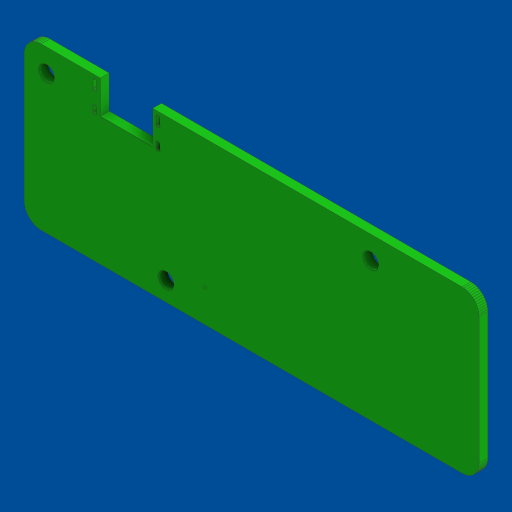
# Autodesk Inventor part: PCB
Saved by Autodesk Inventor 2023.2 (Build 272271000, 271)
## iProperties
Created: 2023-06-14
Part Number: PCB
Material: Generic
Document SubType Name: Modeling
Designer: samdi
Density: 1 g/cm^3
Appearance: Default
Author: samdi
Autodesk Inventor part; units mm, degrees
ref_plane "YZ Plane" through (0, 0, 0) normal (1, 0, 0) x (0, 1, 0)
ref_plane "XZ Plane" through (0, 0, 0) normal (0, 1, 0) x (-1, 0, 0)
ref_plane "XY Plane" through (0, 0, 0) normal (0, 0, 1) x (1, 0, 0)
sketch "Sketch1" plane through (0, 0, 0) normal (0, 0, 1) x (1, 0, 0)
  line L0 (-1.2818, 20.3685) -> (-1.1938, 20.3021)
  line L1 (-1.3879, 20.3987) -> (-1.2818, 20.3685)
  line L2 (-1.4976, 20.3885) -> (-1.3879, 20.3987)
  line L3 (-1.5963, 20.3394) -> (-1.4976, 20.3885)
  line L4 (-1.6706, 20.2579) -> (-1.5963, 20.3394)
  line L5 (-1.1938, 20.3021) -> (-1.1358, 20.2084)
  line L6 (-1.1605, 19.1421) -> (-1.2348, 19.0606)
  line L7 (-1.2348, 19.0606) -> (-1.3335, 19.0115)
  circle A0 centre (6.8571, 2.31) radius 0.15
  circle A1 centre (0, 0) radius 1.35
  line L8 (-1.1156, 19.3) -> (-1.1207, 19.2449)
  line L9 (-1.1156, 20.1) -> (-1.1156, 19.3)
  line L10 (-1.1358, 20.2084) -> (-1.1156, 20.1)
  line L11 (-1.1938, 20.3021) -> (-1.1358, 20.2084)
  line L12 (-1.2818, 20.3685) -> (-1.1938, 20.3021)
  line L13 (-1.3879, 20.3987) -> (-1.2818, 20.3685)
  line L14 (-1.1207, 19.2449) -> (-1.1605, 19.1421)
  circle A2 centre (6.8571, 2.31) radius 0.15
  circle A3 centre (-21, 21) radius 1.35
  line L15 (-22.6676, 24.9248) -> (-22.3359, 24.9811)
  line L16 (-1.1361, 24.2084) -> (-1.1159, 24.1)
  line L17 (-1.7159, 24.1) -> (-1.7107, 24.1551)
  line L18 (-1.7159, 22.9) -> (-1.7159, 24.1)
  line L19 (-1.6956, 22.7916) -> (-1.7159, 22.9)
  line L20 (-1.6376, 22.6979) -> (-1.6956, 22.7916)
  line L21 (-1.1159, 24.1) -> (-1.1159, 22.9)
  line L22 (-1.1159, 22.9) -> (-1.121, 22.8449)
  line L23 (-1.121, 22.8449) -> (-1.1608, 22.7421)
  line L24 (-1.7107, 24.1551) -> (-1.6709, 24.2579)
  line L25 (-1.1941, 24.3021) -> (-1.1361, 24.2084)
  line L26 (-1.2821, 24.3685) -> (-1.1941, 24.3021)
  line L27 (-1.3882, 24.3987) -> (-1.2821, 24.3685)
  line L28 (-1.4979, 24.3885) -> (-1.3882, 24.3987)
  line L29 (-1.5966, 24.3394) -> (-1.4979, 24.3885)
  line L30 (-24.7029, -1.6803) -> (-24.8316, -1.3695)
  line L31 (-24.8316, -1.3695) -> (-24.9248, -1.0462)
  line L32 (-24.9248, -1.0462) -> (-24.9811, -0.7146)
  line L33 (-24.9811, -0.7146) -> (-25, -0.3787)
  line L34 (-25, -0.3787) -> (-25, 22)
  line L35 (-25, 22) -> (-24.9811, 22.3359)
  line L36 (-24.9811, 22.3359) -> (-24.9248, 22.6676)
  line L37 (-24.5402, -1.9748) -> (-24.7029, -1.6803)
  line L38 (-22.9908, 24.8316) -> (-22.6676, 24.9248)
  line L39 (-23.3017, 24.7029) -> (-22.9908, 24.8316)
  line L40 (-23.5961, 24.5402) -> (-23.3017, 24.7029)
  line L41 (-23.8705, 24.3455) -> (-23.5961, 24.5402)
  line L42 (-24.1213, 24.1213) -> (-23.8705, 24.3455)
  line L43 (-24.3455, 23.8705) -> (-24.1213, 24.1213)
  line L44 (-24.5402, 23.5961) -> (-24.3455, 23.8705)
  line L45 (-24.7029, 23.3017) -> (-24.5402, 23.5961)
  line L46 (-24.8316, 22.9908) -> (-24.7029, 23.3017)
  line L47 (-24.9248, 22.6676) -> (-24.8316, 22.9908)
  line L48 (-12.8462, 22.7916) -> (-12.8665, 22.9)
  line L49 (-12.2665, 22.9) -> (-12.2716, 22.8449)
  line L50 (-12.8665, 22.9) -> (-12.8665, 24.1)
  line L51 (-12.2665, 24.1) -> (-12.2665, 22.9)
  line L52 (-12.8665, 24.1) -> (-12.8613, 24.1551)
  line L53 (-12.2867, 24.2084) -> (-12.2665, 24.1)
  line L54 (-12.8613, 24.1551) -> (-12.8215, 24.2579)
  line L55 (-12.3447, 24.3021) -> (-12.2867, 24.2084)
  line L56 (-12.8215, 24.2579) -> (-12.7472, 24.3394)
  line L57 (-12.4327, 24.3685) -> (-12.3447, 24.3021)
  line L58 (-12.5388, 24.3987) -> (-12.4327, 24.3685)
  line L59 (-12.6485, 24.3885) -> (-12.5388, 24.3987)
  line L60 (-12.7472, 24.3394) -> (-12.6485, 24.3885)
  line L61 (-12.2716, 22.8449) -> (-12.3114, 22.7421)
  line L62 (-12.7882, 22.6979) -> (-12.8462, 22.7916)
  line L63 (-12.3114, 22.7421) -> (-12.3857, 22.6606)
  line L64 (-12.7002, 22.6315) -> (-12.7882, 22.6979)
  line L65 (-12.3857, 22.6606) -> (-12.4844, 22.6115)
  line L66 (-12.5941, 22.6013) -> (-12.7002, 22.6315)
  line L67 (-12.4844, 22.6115) -> (-12.5941, 22.6013)
  line L68 (-1.7104, 20.1551) -> (-1.6706, 20.2579)
  line L69 (-1.7156, 20.1) -> (-1.7104, 20.1551)
  line L70 (-1.5493, 19.0315) -> (-1.6373, 19.0979)
  line L71 (-1.7156, 19.3) -> (-1.7156, 20.1)
  line L72 (-1.6953, 19.1916) -> (-1.7156, 19.3)
  line L73 (-1.6373, 19.0979) -> (-1.6953, 19.1916)
  line L74 (-1.1605, 19.1421) -> (-1.2348, 19.0606)
  line L75 (-1.2348, 19.0606) -> (-1.3335, 19.0115)
  line L76 (-1.3335, 19.0115) -> (-1.4432, 19.0013)
  line L77 (-1.4432, 19.0013) -> (-1.5493, 19.0315)
  line L78 (-1.1207, 19.2449) -> (-1.1605, 19.1421)
  line L79 (-1.1608, 22.7421) -> (-1.2351, 22.6606)
  line L80 (-1.2351, 22.6606) -> (-1.3338, 22.6115)
  line L81 (-1.3338, 22.6115) -> (-1.4435, 22.6013)
  line L82 (-1.4435, 22.6013) -> (-1.5496, 22.6315)
  line L83 (-1.5496, 22.6315) -> (-1.6376, 22.6979)
  line L84 (-1.1159, 24.1) -> (-1.1159, 22.9)
  line L85 (-1.1159, 22.9) -> (-1.121, 22.8449)
  line L86 (-1.1361, 24.2084) -> (-1.1159, 24.1)
  line L87 (-1.121, 22.8449) -> (-1.1608, 22.7421)
  line L88 (-1.1941, 24.3021) -> (-1.1361, 24.2084)
  line L89 (-1.2821, 24.3685) -> (-1.1941, 24.3021)
  line L90 (-1.3335, 19.0115) -> (-1.4432, 19.0013)
  line L91 (-1.4979, 24.3885) -> (-1.3882, 24.3987)
  line L92 (-1.5966, 24.3394) -> (-1.4979, 24.3885)
  line L93 (-1.6709, 24.2579) -> (-1.5966, 24.3394)
  line L94 (-1.3882, 24.3987) -> (-1.2821, 24.3685)
  line L95 (-1.4976, 20.3885) -> (-1.3879, 20.3987)
  line L96 (-1.5963, 20.3394) -> (-1.4976, 20.3885)
  line L97 (-1.4432, 19.0013) -> (-1.5493, 19.0315)
  line L98 (-1.6706, 20.2579) -> (-1.5963, 20.3394)
  line L99 (-1.7104, 20.1551) -> (-1.6706, 20.2579)
  line L100 (-1.5493, 19.0315) -> (-1.6373, 19.0979)
  line L101 (-1.6373, 19.0979) -> (-1.6953, 19.1916)
  line L102 (-1.7156, 19.3) -> (-1.7156, 20.1)
  line L103 (-1.6953, 19.1916) -> (-1.7156, 19.3)
  line L104 (-1.7156, 20.1) -> (-1.7104, 20.1551)
  line L105 (-1.6956, 22.7916) -> (-1.7159, 22.9)
  line L106 (-1.6709, 24.2579) -> (-1.5966, 24.3394)
  line L107 (-1.5496, 22.6315) -> (-1.6376, 22.6979)
  line L108 (-1.4435, 22.6013) -> (-1.5496, 22.6315)
  line L109 (-1.3338, 22.6115) -> (-1.4435, 22.6013)
  line L110 (-1.2351, 22.6606) -> (-1.3338, 22.6115)
  line L111 (-1.1608, 22.7421) -> (-1.2351, 22.6606)
  line L112 (-1.1156, 19.3) -> (-1.1207, 19.2449)
  line L113 (-1.1156, 20.1) -> (-1.1156, 19.3)
  line L114 (-1.1358, 20.2084) -> (-1.1156, 20.1)
  line L115 (-2.3912, 25) -> (1.7088, 25)
  circle A4 centre (0, 0) radius 1.35
  line L116 (-12.8215, 20.2579) -> (-12.7472, 20.3394)
  line L117 (-12.8613, 20.1551) -> (-12.8215, 20.2579)
  line L118 (-2.3912, 25) -> (1.7088, 25)
  line L119 (-2.3912, 19.2) -> (-2.3912, 25)
  line L120 (-2.3912, 19.2) -> (-2.3912, 25)
  line L121 (-11.5911, 19.2) -> (-2.3912, 19.2)
  line L122 (-11.5911, 19.2) -> (-2.3912, 19.2)
  line L123 (-11.5911, 25) -> (-11.5911, 19.2)
  line L124 (-11.5911, 25) -> (-11.5911, 19.2)
  line L125 (-12.7472, 24.3394) -> (-12.6485, 24.3885)
  line L126 (-12.3114, 22.7421) -> (-12.3857, 22.6606)
  line L127 (-12.3857, 22.6606) -> (-12.4844, 22.6115)
  line L128 (-12.4844, 22.6115) -> (-12.5941, 22.6013)
  line L129 (-12.5941, 22.6013) -> (-12.7002, 22.6315)
  line L130 (-12.7002, 22.6315) -> (-12.7882, 22.6979)
  line L131 (-12.7882, 22.6979) -> (-12.8462, 22.7916)
  line L132 (-12.8462, 22.7916) -> (-12.8665, 22.9)
  line L133 (-12.8665, 22.9) -> (-12.8665, 24.1)
  line L134 (-12.8665, 24.1) -> (-12.8613, 24.1551)
  line L135 (-12.8613, 24.1551) -> (-12.8215, 24.2579)
  line L136 (-12.2867, 24.2084) -> (-12.2665, 24.1)
  line L137 (-12.2665, 24.1) -> (-12.2665, 22.9)
  line L138 (-12.2665, 22.9) -> (-12.2716, 22.8449)
  line L139 (-12.2716, 22.8449) -> (-12.3114, 22.7421)
  line L140 (-12.8462, 19.1916) -> (-12.8665, 19.3)
  line L141 (-12.8665, 19.3) -> (-12.8665, 20.1)
  line L142 (-1.7107, 24.1551) -> (-1.6709, 24.2579)
  line L143 (-1.7159, 24.1) -> (-1.7107, 24.1551)
  line L144 (-1.7159, 22.9) -> (-1.7159, 24.1)
  line L145 (-1.6376, 22.6979) -> (-1.6956, 22.7916)
  line L146 (-12.2867, 20.2084) -> (-12.2665, 20.1)
  line L147 (-12.2665, 20.1) -> (-12.2665, 19.3)
  line L148 (-12.3447, 20.3021) -> (-12.2867, 20.2084)
  line L149 (-12.2665, 19.3) -> (-12.2716, 19.2449)
  line L150 (-12.2716, 19.2449) -> (-12.3114, 19.1421)
  line L151 (-12.4327, 20.3685) -> (-12.3447, 20.3021)
  line L152 (-12.5388, 20.3987) -> (-12.4327, 20.3685)
  line L153 (-12.6485, 20.3885) -> (-12.5388, 20.3987)
  line L154 (-12.8665, 20.1) -> (-12.8613, 20.1551)
  line L155 (-12.7472, 20.3394) -> (-12.6485, 20.3885)
  line L156 (-12.6485, 20.3885) -> (-12.5388, 20.3987)
  line L157 (-12.7472, 20.3394) -> (-12.6485, 20.3885)
  line L158 (-12.4327, 20.3685) -> (-12.3447, 20.3021)
  line L159 (-12.8215, 20.2579) -> (-12.7472, 20.3394)
  line L160 (-12.3447, 20.3021) -> (-12.2867, 20.2084)
  line L161 (-12.8613, 20.1551) -> (-12.8215, 20.2579)
  line L162 (-12.2867, 20.2084) -> (-12.2665, 20.1)
  line L163 (-12.8665, 20.1) -> (-12.8613, 20.1551)
  line L164 (-12.8665, 19.3) -> (-12.8665, 20.1)
  line L165 (-12.2665, 20.1) -> (-12.2665, 19.3)
  line L166 (-12.2665, 19.3) -> (-12.2716, 19.2449)
  line L167 (-12.5388, 20.3987) -> (-12.4327, 20.3685)
  line L168 (-12.8462, 19.1916) -> (-12.8665, 19.3)
  line L169 (-12.7882, 19.0979) -> (-12.8462, 19.1916)
  line L170 (-12.7002, 19.0315) -> (-12.7882, 19.0979)
  line L171 (-12.5941, 19.0013) -> (-12.7002, 19.0315)
  line L172 (-12.4844, 19.0115) -> (-12.5941, 19.0013)
  line L173 (-12.3857, 19.0606) -> (-12.4844, 19.0115)
  line L174 (-12.3114, 19.1421) -> (-12.3857, 19.0606)
  line L175 (-12.2716, 19.2449) -> (-12.3114, 19.1421)
  line L176 (-15.0912, 25) -> (-11.5911, 25)
  line L177 (-22, 25) -> (-15.0912, 25)
  line L178 (-22.3359, 24.9811) -> (-22, 25)
  line L179 (-12.3447, 24.3021) -> (-12.2867, 24.2084)
  line L180 (-12.3114, 19.1421) -> (-12.3857, 19.0606)
  line L181 (-12.4327, 24.3685) -> (-12.3447, 24.3021)
  line L182 (-12.3857, 19.0606) -> (-12.4844, 19.0115)
  line L183 (-12.4844, 19.0115) -> (-12.5941, 19.0013)
  line L184 (-12.6485, 24.3885) -> (-12.5388, 24.3987)
  line L185 (-12.5941, 19.0013) -> (-12.7002, 19.0315)
  line L186 (-12.7002, 19.0315) -> (-12.7882, 19.0979)
  line L187 (-12.7882, 19.0979) -> (-12.8462, 19.1916)
  line L188 (-12.8215, 24.2579) -> (-12.7472, 24.3394)
  line L189 (-15.0912, 25) -> (-11.5911, 25)
  line L190 (-22, 25) -> (-15.0912, 25)
  circle A5 centre (-21, 21) radius 1.35
  line L191 (-12.5388, 24.3987) -> (-12.4327, 24.3685)
  line L192 (-22.3359, 24.9811) -> (-22, 25)
  line L193 (-22.6676, 24.9248) -> (-22.3359, 24.9811)
  line L194 (-22.9908, 24.8316) -> (-22.6676, 24.9248)
  line L195 (-23.5961, 24.5402) -> (-23.3017, 24.7029)
  line L196 (-23.3017, 24.7029) -> (-22.9908, 24.8316)
  line L197 (-23.8705, 24.3455) -> (-23.5961, 24.5402)
  line L198 (-24.1213, 24.1213) -> (-23.8705, 24.3455)
  line L199 (-24.5402, 23.5961) -> (-24.3455, 23.8705)
  line L200 (-24.7029, 23.3017) -> (-24.5402, 23.5961)
  line L201 (-24.3455, 23.8705) -> (-24.1213, 24.1213)
  line L202 (-25, -0.3787) -> (-25, 22)
  line L203 (-25, 22) -> (-24.9811, 22.3359)
  line L204 (-24.9811, 22.3359) -> (-24.9248, 22.6676)
  line L205 (-24.8316, 22.9908) -> (-24.7029, 23.3017)
  line L206 (-24.9248, 22.6676) -> (-24.8316, 22.9908)
  line L207 (-23.3017, -3.0816) -> (-23.5961, -2.9189)
  line L208 (-23.5961, -2.9189) -> (-23.8705, -2.7242)
  line L209 (-23.8705, -2.7242) -> (-24.1213, -2.5)
  line L210 (-24.1213, -2.5) -> (-24.3455, -2.2491)
  line L211 (-24.3455, -2.2491) -> (-24.5402, -1.9748)
  line L212 (-24.3455, -2.2491) -> (-24.5402, -1.9748)
  line L213 (-24.1213, -2.5) -> (-24.3455, -2.2491)
  line L214 (-23.8705, -2.7242) -> (-24.1213, -2.5)
  line L215 (52, -3.3787) -> (-22, -3.3787)
  line L216 (52, -3.3787) -> (-22, -3.3787)
  line L217 (1.7088, 25) -> (52, 25)
  line L218 (1.7088, 25) -> (52, 25)
  circle A6 centre (36, 21) radius 1.35
  line L219 (52, 25) -> (52.3359, 24.9811)
  line L220 (52.6676, 24.9248) -> (52.9908, 24.8316)
  line L221 (52.9908, 24.8316) -> (53.3017, 24.7029)
  line L222 (53.8705, 24.3455) -> (54.1213, 24.1213)
  line L223 (54.3455, 23.8705) -> (54.5402, 23.5961)
  line L224 (54.8317, 22.9908) -> (54.9248, 22.6676)
  line L225 (54.8317, 22.9908) -> (54.9248, 22.6676)
  line L226 (52.3359, -3.3598) -> (52, -3.3787)
  line L227 (52, 25) -> (52.3359, 24.9811)
  line L228 (52.3359, 24.9811) -> (52.6676, 24.9248)
  line L229 (52.3359, 24.9811) -> (52.6676, 24.9248)
  line L230 (52.6676, 24.9248) -> (52.9908, 24.8316)
  line L231 (53.3017, 24.7029) -> (53.5961, 24.5402)
  line L232 (53.3017, 24.7029) -> (53.5961, 24.5402)
  line L233 (53.5961, 24.5402) -> (53.8705, 24.3455)
  line L234 (54.9811, 22.3359) -> (55, 22)
  line L235 (54.1213, 24.1213) -> (54.3455, 23.8705)
  line L236 (54.9248, 22.6676) -> (54.9811, 22.3359)
  line L237 (54.5402, 23.5961) -> (54.7029, 23.3017)
  line L238 (54.7029, 23.3017) -> (54.8317, 22.9908)
  line L239 (52.9908, 24.8316) -> (53.3017, 24.7029)
  line L240 (53.5961, 24.5402) -> (53.8705, 24.3455)
  line L241 (55, 22) -> (55, -0.3787)
  line L242 (53.5961, -2.9189) -> (53.3017, -3.0816)
  line L243 (53.5961, -2.9189) -> (53.3017, -3.0816)
  line L244 (54.3455, -2.2491) -> (54.1213, -2.5)
  line L245 (54.8317, -1.3695) -> (54.7029, -1.6803)
  line L246 (54.9811, -0.7146) -> (54.9248, -1.0462)
  line L247 (54.9248, -1.0462) -> (54.8317, -1.3695)
  line L248 (54.7029, -1.6803) -> (54.5402, -1.9748)
  line L249 (54.5402, -1.9748) -> (54.3455, -2.2491)
  line L250 (54.1213, -2.5) -> (53.8705, -2.7242)
  line L251 (53.3017, -3.0816) -> (52.9908, -3.2103)
  line L252 (52.9908, -3.2103) -> (52.6676, -3.3035)
  line L253 (52.3359, -3.3598) -> (52, -3.3787)
  line L254 (55, -0.3787) -> (54.9811, -0.7146)
  line L255 (-22, -3.3787) -> (-22.3359, -3.3598)
  line L256 (-22.6676, -3.3035) -> (-22.9908, -3.2103)
  line L257 (-22.9908, -3.2103) -> (-23.3017, -3.0816)
  line L258 (-22.3359, -3.3598) -> (-22.6676, -3.3035)
  line L259 (-22, -3.3787) -> (-22.3359, -3.3598)
  line L260 (-23.5961, -2.9189) -> (-23.8705, -2.7242)
  line L261 (-23.3017, -3.0816) -> (-23.5961, -2.9189)
  line L262 (-22.9908, -3.2103) -> (-23.3017, -3.0816)
  line L263 (-22.6676, -3.3035) -> (-22.9908, -3.2103)
  line L264 (-22.3359, -3.3598) -> (-22.6676, -3.3035)
  circle A7 centre (36, 21) radius 1.35
  line L265 (52.6676, -3.3035) -> (52.3359, -3.3598)
  line L266 (53.3017, -3.0816) -> (52.9908, -3.2103)
  line L267 (53.8705, -2.7242) -> (53.5961, -2.9189)
  line L268 (55, -0.3787) -> (54.9811, -0.7146)
  line L269 (54.7029, -1.6803) -> (54.5402, -1.9748)
  line L270 (52.6676, -3.3035) -> (52.3359, -3.3598)
  line L271 (53.8705, 24.3455) -> (54.1213, 24.1213)
  line L272 (54.1213, 24.1213) -> (54.3455, 23.8705)
  line L273 (54.3455, 23.8705) -> (54.5402, 23.5961)
  line L274 (54.5402, 23.5961) -> (54.7029, 23.3017)
  line L275 (54.7029, 23.3017) -> (54.8317, 22.9908)
  line L276 (54.9248, 22.6676) -> (54.9811, 22.3359)
  line L277 (54.9811, 22.3359) -> (55, 22)
  line L278 (55, 22) -> (55, -0.3787)
  line L279 (52.9908, -3.2103) -> (52.6676, -3.3035)
  line L280 (53.8705, -2.7242) -> (53.5961, -2.9189)
  line L281 (54.1213, -2.5) -> (53.8705, -2.7242)
  line L282 (54.3455, -2.2491) -> (54.1213, -2.5)
  line L283 (54.5402, -1.9748) -> (54.3455, -2.2491)
  line L284 (54.9811, -0.7146) -> (54.9248, -1.0462)
  line L285 (54.9248, -1.0462) -> (54.8317, -1.3695)
  line L286 (54.8317, -1.3695) -> (54.7029, -1.6803)
  line L287 (-24.5402, -1.9748) -> (-24.7029, -1.6803)
  line L288 (-24.7029, -1.6803) -> (-24.8316, -1.3695)
  line L289 (-24.8316, -1.3695) -> (-24.9248, -1.0462)
  line L290 (-24.9248, -1.0462) -> (-24.9811, -0.7146)
  line L291 (-24.9811, -0.7146) -> (-25, -0.3787)
  constraints: 584 end point, 8 centre point
extrude "Extrusion1" add sketch "Sketch1" along normal blind 1.55
body "Solid1"
